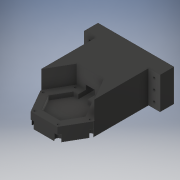
# Autodesk Inventor part: TARM01
Saved by Autodesk Inventor 2017 (Build 210142000, 142)
## iProperties
Created: 2018-10-11
Part Number: TARM01
Material: ABS Plastic
Document SubType Name: Modeling
Designer: Zach
Density: 1.06 g/cm^3
Appearance: Smooth - Black
Author: Zach
Autodesk Inventor part; units mm, degrees
ref_plane "YZ Plane" through (0, 0, 0) normal (1, 0, 0) x (0, 1, 0)
ref_plane "XZ Plane" through (0, 0, 0) normal (0, 1, 0) x (-1, 0, 0)
ref_plane "XY Plane" through (0, 0, 0) normal (0, 0, 1) x (1, 0, 0)
sketch "Sketch24" plane through (0, 0, 0) normal (0, 0, 1) x (1, 0, 0)
  line L0 (0, 0) -> (165, 0)
  line L1 (165, 0) -> (165, 70)
  line L2 (165, 70) -> (0, 70)
  line L3 (0, 70) -> (0, 0)
  circle A0 centre (12.5, 57.5) radius 2.5
  circle A1 centre (12.5, 35) radius 2.5
  circle A2 centre (12.5, 12.5) radius 2.5
  line L4 (12.5, 57.5) -> (12.5, 12.5) construction
  line L5 (82.5, 70) -> (82.5, 0) construction
  circle A3 centre (152.5, 57.5) radius 2.5
  circle A4 centre (152.5, 35) radius 2.5
  circle A5 centre (152.5, 12.5) radius 2.5
  line L6 (152.5, 57.5) -> (152.5, 12.5) construction
  point P0 (0, 35)
  dimension "d100" = 165
  dimension "d101" = 70
  dimension "d102" = 5
  dimension "d103" = 5
  dimension "d104" = 5
  dimension "d105" = 45
  dimension "d106" = 12.5
  constraints: 14 end point, 6 centre point, 4 midpoint, 4 symmetric about line, 2 coincident, 2 parallel, 1 horizontal, 1 horizontal alignment, 1 perpendicular, 1 vertical, 3 other
  measures "d100" distance of L2.end L1.end
  measures "d101" distance of L1.end L0.end
  measures "d102" diameter of A0
  measures "d103" diameter of A1
  measures "d104" diameter of A2
  measures "d105" distance of L4.start L4.end
  measures "d106" distance between parallel lines of L3 L4
extrude "Extrusion21" add sketch "Sketch24" along normal blind 30
sketch "Sketch25" plane through (0, 0, 30) normal (0, 0, 1) x (1, 0, 0)
  line L0 (165, 70) -> (0, 70) projected
  line L1 (0, 0) -> (165, 0) projected
  line L2 (25, 70) -> (140, 70)
  line L3 (140, 70) -> (140, 0)
  line L4 (140, 0) -> (25, 0)
  line L5 (25, 0) -> (25, 70)
  point P0 (82.5, 70)
  dimension "d109" = 115
  constraints: 8 end point, 2 midpoint, 2 parallel, 2 point on line, 1 horizontal, 1 perpendicular
  measures "d109" distance between parallel lines of L3 L5
extrude "Extrusion22" add sketch "Sketch25" along normal blind 170
sketch "Sketch26" plane through (0, 70, 0) normal (0, 1, 0) x (1, 0, 0)
  line L0 (25, -30) -> (25, -200) projected
  line L1 (25, -150.2035) -> (53.75, -100.4071)
  line L2 (53.75, -100.4071) -> (111.25, -100.4071)
  line L3 (111.25, -100.4071) -> (140, -150.2035)
  line L4 (140, -150.2035) -> (111.25, -200)
  line L5 (111.25, -200) -> (53.75, -200)
  line L6 (53.75, -200) -> (25, -150.2035)
  line L7 (140, -30) -> (140, -200) projected
  line L8 (140, -200) -> (25, -200) projected
  point P0 (0, 0)
  point P1 (82.5, -150.2035)
  point P2 (82.5, -200)
  constraints: 12 end point, 2 midpoint, 2 point on line, 1 horizontal alignment, 13 other
extrude "Extrusion23" cut sketch "Sketch26" against normal through all contours L6 L8 L0 | L4 L7 L8
sketch "Sketch27" plane through (0, 70, 0) normal (0, 1, 0) x (1, 0, 0)
  line L0 (25, -150.2035) -> (53.75, -200) projected
  line L1 (111.25, -200) -> (53.75, -200) projected
  line L2 (111.25, -200) -> (140, -150.2035) projected
  line L3 (53.75, -200) -> (25, -150.2035)
  line L4 (25, -150.2035) -> (53.75, -100.4071)
  line L5 (53.75, -100.4071) -> (111.25, -100.4071)
  line L6 (111.25, -100.4071) -> (140, -150.2035)
  line L7 (140, -150.2035) -> (111.25, -200)
  line L8 (111.25, -200) -> (53.75, -200)
  line L9 (53.1726, -99.4071) -> (23.8453, -150.2035)
  line L10 (23.8453, -150.2035) -> (53.1726, -201)
  line L11 (53.1726, -201) -> (111.8274, -201)
  line L12 (111.8274, -201) -> (141.1547, -150.2035)
  line L13 (141.1547, -150.2035) -> (111.8274, -99.4071)
  line L14 (111.8274, -99.4071) -> (53.1726, -99.4071)
  point P0 (0, 0)
  point P1 (82.5, -150.2035)
  dimension "d114" = 1
  constraints: 24 end point, 18 other
  measures "d114" distance between parallel lines of L4 L9
extrude "Extrusion24" cut sketch "Sketch27" against normal blind 40 contours L4 L5 L6 L2 L1 L0 | L14 L13 L12 L11 L10 L9
sketch "Sketch28" plane through (0, 30, 0) normal (0, 1, 0) x (1, 0, 0)
  circle A0 centre (31.5, -150.2035) radius 2.5
  line L0 (53.75, -200) -> (25, -150.2035) projected
  line L1 (140, -148.2035) -> (140, -150.2035) construction
  line L2 (25, -150.2035) -> (140, -150.2035) construction
  circle A1 centre (82.5, -150.2035) radius 2.5 construction
  circle A2 centre (133.5, -150.2035) radius 2.5 construction
  line L3 (31.5, -150.2035) -> (133.5, -150.2035) construction
  circle A3 centre (57, -194.3708) radius 2.5
  circle A4 centre (108, -194.3708) radius 2.5
  circle A5 centre (133.5, -150.2035) radius 2.5
  circle A6 centre (108, -106.0362) radius 2.5
  circle A7 centre (57, -106.0362) radius 2.5
  point P0 (0, 0)
  dimension "d117" = 5
  dimension "d118" = 5
  dimension "d119" = 5
  dimension "d120" = 102
  dimension "d123" = 360
  constraints: 8 centre point, 4 end point, 2 horizontal, 2 midpoint, 2 point on line, 13 other
  measures "d117" diameter of A0
  measures "d118" diameter of A1
  measures "d119" diameter of A2
  measures "d120" distance of L3.end L3.start
extrude "Extrusion25" cut sketch "Sketch28" against normal through all
sketch "Sketch29" plane through (0, 0, 0) normal (0, -1, 0) x (1, 0, 0)
  circle A0 centre (57, 194.3708) radius 2.5 construction
  circle A1 centre (108, 106.0362) radius 2.5 construction
  line L0 (57, 194.3708) -> (108, 106.0362) construction
  circle A2 centre (57, 194.3708) radius 6.5
  line L1 (31.5, 150.2035) -> (133.5, 150.2035) construction
  circle A3 centre (31.5, 150.2035) radius 6.5
  line L2 (57, 106.0362) -> (108, 194.3708) construction
  circle A4 centre (57, 106.0362) radius 6.5
  line L3 (108, 106.0362) -> (57, 194.3708) construction
  circle A5 centre (108, 106.0362) radius 6.5
  line L4 (133.5, 150.2035) -> (31.5, 150.2035) construction
  circle A6 centre (133.5, 150.2035) radius 6.5
  line L5 (108, 194.3708) -> (57, 106.0362) construction
  circle A7 centre (108, 194.3708) radius 6.5
  point P0 (0, 0)
  point P1 (82.5, 150.2035)
  point P2 (82.5, 150.2035)
  point P3 (82.5, 150.2035)
  point P4 (82.5, 150.2035)
  point P5 (82.5, 150.2035)
  point P6 (82.5, 150.2035)
  dimension "d127" = 13
  dimension "d130" = 360
  constraints: 12 end point, 8 coincident, 6 centre point, 1 midpoint, 35 other
  measures "d127" diameter of A2
extrude "Extrusion26" cut sketch "Sketch29" against normal blind 15
sketch "Sketch30" plane through (0, 30, 0) normal (0, 1, 0) x (1, 0, 0)
  line L0 (53.75, -200) -> (25, -150.2035) construction
  line L1 (111.25, -200) -> (53.75, -200) construction
  line L2 (140, -150.2035) -> (111.25, -200) construction
  circle A0 centre (133.5, -150.2035) radius 2.5 construction
  circle A1 centre (31.5, -150.2035) radius 2.5 construction
  circle A2 centre (133.5, -150.2035) radius 2.5 construction
  line L3 (31.5, -150.2035) -> (133.5, -150.2035) construction
  line L4 (102.5897, -185) -> (62.4103, -185)
  line L5 (62.4103, -185) -> (42.3205, -150.2035)
  line L6 (42.3205, -150.2035) -> (62.4103, -115.4071)
  line L7 (62.4103, -115.4071) -> (102.5897, -115.4071)
  line L8 (102.5897, -115.4071) -> (122.6795, -150.2035)
  line L9 (122.6795, -150.2035) -> (102.5897, -185)
  point P0 (0, 0)
  point P1 (82.5, -150.2035)
  point P2 (82.5, -150.2035)
  dimension "d134" = 15
  constraints: 14 end point, 1 coincident, 1 horizontal, 1 midpoint, 1 point on line, 13 other
  measures "d134" distance between parallel lines of L1 L4
extrude "Extrusion27" cut sketch "Sketch30" against normal blind 10
sketch "Sketch31" plane through (62.4103, 30, 115.4071) normal (0, 0, 1) x (1, 0, 0)
  line L0 (-9.2376, 40) -> (49.4171, 40) projected
  line L1 (-9.2376, 40) -> (-9.2376, 0) projected
  line L2 (-9.2376, 0) -> (49.4171, 0) projected
  line L3 (49.4171, 40) -> (49.4171, 0) projected
  line L4 (0, 0) -> (40.1795, 0) projected
  line L5 (0, 0) -> (0, -10) projected
  line L6 (0, -10) -> (40.1795, -10) projected
  line L7 (40.1795, 0) -> (40.1795, -10) projected
  line L8 (10.0897, -10) -> (30.0897, -10)
  line L9 (30.0897, -10) -> (30.0897, 10)
  line L10 (30.0897, 10) -> (10.0897, 10)
  line L11 (10.0897, 10) -> (10.0897, -10)
  point P0 (-62.4103, -30)
  point P1 (20.0897, -10)
  dimension "d137" = 20
  dimension "d138" = 20
  constraints: 8 end point, 2 midpoint, 2 parallel, 1 horizontal, 1 perpendicular, 1 point on line
  measures "d137" distance of L9.end L10.end
  measures "d138" distance of L10.end L8.start
extrude "Extrusion28" cut sketch "Sketch31" against normal through all contours L11 L10 L9 L2 | L2 L9 L6 L11
body "Solid3"
